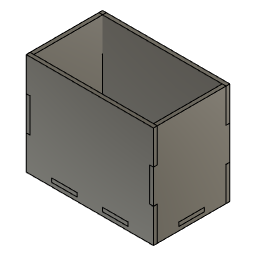
Parametric Box (Autodesk Fusion 360 design; units mm, degrees)
Autodesk Fusion 360 part; units mm, degrees
sketch "Sketch1" plane through (0, 0, 0) normal (0, 1, 0) x (1, 0, 0) in component "front"
  line L0 (0, 0) -> (100, 0)
  line L1 (100, 0) -> (100, -80)
  line L2 (100, -80) -> (0, -80)
  line L3 (0, -80) -> (0, 0)
  line L4 (3, 0) -> (3, -80) construction
  line L5 (0, -6) -> (100, -6) construction
  line L6 (100, -3) -> (0, -3) construction
  line L7 (50, -80) -> (50, 0) construction
  line L8 (20, -6) -> (40, -6)
  line L9 (40, -6) -> (40, -3)
  line L10 (40, -3) -> (20, -3)
  line L11 (20, -3) -> (20, -6)
  line L12 (60, -6) -> (80, -6)
  line L13 (80, -6) -> (80, -3)
  line L14 (80, -3) -> (60, -3)
  line L15 (60, -3) -> (60, -6)
  line L16 (0, -53.3333) -> (3, -53.3333)
  line L17 (3, -53.3333) -> (3, -26.6667)
  line L18 (3, -26.6667) -> (0, -26.6667)
  line L19 (0, -26.6667) -> (0, -53.3333)
  line L20 (100, -53.3333) -> (97, -53.3333)
  line L21 (100, -80) -> (100, 0)
  line L22 (97, -26.6667) -> (100, -26.6667)
  line L23 (97, 0) -> (97, -80) construction
  line L24 (100, -26.6667) -> (100, -53.3333)
  line L25 (97, -53.3333) -> (97, -26.6667)
  dimension "d10" = 100
  dimension "d11" = 80
  dimension "d12" = 3
  dimension "d13" = 3
  dimension "d14" = 3
  dimension "d17" = 20
  dimension "d18" = 20
  dimension "d19" = 20
  dimension "d20" = 20
  dimension "d21" = 26.6667
  dimension "d22" = 26.6667
  constraint horizontal L0
  constraint vertical L1
  constraint horizontal L2
  constraint vertical L3
  constraint coincident L0.start L3.end
  constraint coincident L0 L4.start
  constraint coincident L2 L4.end
  constraint perpendicular L2 L4
  constraint coincident L3 L5.start
  constraint coincident L1 L5.end
  constraint perpendicular L1 L5
  constraint coincident L1 L6.start
  constraint perpendicular L3 L6
  constraint coincident L3 L6.end
  constraint midpoint L2 L7.start
  constraint perpendicular L5 L7
  constraint horizontal L8
  constraint vertical L9
  constraint horizontal L10
  constraint vertical L11
  constraint coincident L6 L9.end
  constraint coincident L5 L8.start
  constraint horizontal L12
  constraint vertical L13
  constraint horizontal L14
  constraint vertical L15
  constraint coincident L6 L13.end
  constraint coincident L5 L12.start
  constraint horizontal L16
  constraint vertical L17
  constraint horizontal L18
  constraint vertical L19
  constraint coincident L4 L17.end
  constraint coincident L3 L16.start
  constraint symmetric L0.start L7 L0.end
  constraint symmetric L2.end L7 L1.end
  constraint symmetric L4.start L7 L23.start
  constraint symmetric L4.end L7 L23.end
  constraint symmetric L7 L16.start L20.start
  constraint symmetric L7 L16.end L20.end
  constraint symmetric L7 L17.end L22.start
  constraint symmetric L7 L18.end L22.end
  measures "d10" distance of L0.start L0.end
  measures "d11" distance of L0.start L2.end
  measures "d12" distance of L0 L6
  measures "d13" distance of L5 L6
  measures "d14" distance of L3 L4
  measures "d17" distance of L3 L8.start
  measures "d18" distance of L9.end L10.end
  measures "d19" distance of L9.end L14.end
  measures "d20" distance of L13.end L14.end
  measures "d21" distance of L2 L16
  measures "d22" distance of L16 L18
extrude "Extrude1" add sketch "Sketch1" along normal blind 3 contours L0 L1 L2 L3 L16 L17 L18 L20 L21 L22 L25 makes body 1 in component "front"
sketch "Sketch1 (2)" plane through (0, 0, 0) normal (1, 0, 0) x (0, 1, 0) in component "left"
sketch "Sketch2" plane through (0, 0, 0) normal (1, 0, 0) x (0, 1, 0) in component "left"
  line L0 (0, 0) -> (60, 0)
  line L1 (60, 0) -> (60, 80)
  line L2 (60, 80) -> (0, 80)
  line L3 (0, 80) -> (0, 0)
  line L4 (0, 80) -> (0, 53.3333)
  line L5 (0, 80) -> (3, 80)
  line L6 (0, 0) -> (3, 0)
  line L7 (0, 6) -> (60, 6) construction
  line L8 (0, 3) -> (60, 3) construction
  line L9 (40, 6) -> (20, 6)
  line L10 (20, 6) -> (20, 3)
  line L11 (20, 3) -> (40, 3)
  line L12 (40, 3) -> (40, 6)
  dimension "d25" = 60
  dimension "d26" = 20
  dimension "d27" = 20
  dimension "d28" = 3
  dimension "d29" = 3
  constraint horizontal L0
  constraint vertical L1
  constraint horizontal L2
  constraint vertical L3
  constraint collinear L3 L4
  constraint collinear L2 L5
  constraint collinear L0 L6
  constraint coincident L3 L7.start
  constraint coincident L1 L7.end
  constraint perpendicular L1 L7
  constraint coincident L3 L8.start
  constraint coincident L1 L8.end
  constraint perpendicular L1 L8
  constraint horizontal L9
  constraint vertical L10
  constraint horizontal L11
  constraint vertical L12
  constraint coincident L7 L9.start
  measures "d25" distance of L1 L3
  measures "d26" distance of L9.start L9.end
  measures "d27" distance of L1 L12
  measures "d28" distance of L7 L8
  measures "d29" distance of L0 L8
extrude "Extrude1'" add sketch "Sketch2" along normal blind 3 separate body makes body 2 in component "left"
combine "Combine1" operation cut target body 2 tool bodies 1 keep tools in component "left"
ref_plane "WorkPlane1" through (50, 1.5, 66.6667) normal (-1, 0, 0) x (0, 0, 1)
mirror "MirrorComponent1" about plane through (0, 0, 0) normal (0, 0, 1) of bodies 2 makes body 3 in component "left(Mirror)"
ref_plane "WorkPlane2" through (1.5, 30, 40) normal (0, 1, 0) x (0, 0, 1)
mirror "MirrorComponent2" about plane through (0, 0, 0) normal (0, 0, 1) of bodies 1 makes body 4 in component "front(Mirror)"
combine "Combine1'" operation cut target body 3 tool bodies 4 body 4 seen with x (-1, 0, 0) y (0, -1, 0) z (0, 0, 1) at (100, 60, 0) keep tools in component "left(Mirror)"
ref_plane "WorkPlane1" through (0, 0, 3) normal (0, 0, 1) x (1, 0, 0) in component "base"
sketch "Sketch1 (3)" plane through (0, 0, 3) normal (0, 0, 1) x (1, 0, 0) in component "base"
  line L0 (0, 60) -> (100, 60)
  line L1 (100, 60) -> (100, 0)
  line L2 (100, 0) -> (0, 0)
  line L3 (0, 0) -> (0, 60)
  constraint horizontal L0
  constraint vertical L1
  constraint horizontal L2
  constraint vertical L3
extrude "Extrude1''" add sketch "Sketch1 (3)" along normal blind 3 separate body makes body 5 in component "base"
combine "Combine1''" operation cut target body 5 tool bodies 2 4 3 1 body 4 seen with x (1, 0, 0) y (0, -1, 0) z (0, 0, -1) at (0, 60, 0) body 3 seen with x (-1, 0, 0) y (0, 1, 0) z (0, 0, -1) at (100, 0, 0) keep tools in component "base"
component "front" placed x (1, 0, 0) y (0, 1, 0) z (0, 0, 1) at (0, 0, 0)
component "left" placed x (1, 0, 0) y (0, 1, 0) z (0, 0, 1) at (0, 0, 0)
component "left(Mirror)" placed x (-1, 0, 0) y (0, 1, 0) z (0, 0, -1) at (100, 0, 0)
component "front(Mirror)" placed x (1, 0, 0) y (0, -1, 0) z (0, 0, -1) at (0, 60, 0)
component "base" placed x (1, 0, 0) y (0, 1, 0) z (0, 0, 1) at (0, 0, 0)
equation "length = 100 mm"
equation "width = 60 mm"
equation "height = 80 mm"
equation "thick = 3 mm"
equation "ntabs_L = 5"
equation "ntabs_W = 3"
equation "ntabs_H = 3"
equation "d10 = length"
equation "d11 = height"
equation "d12 = thick"
equation "d13 = thick"
equation "d14 = thick"
equation "d15 = length / ntabs_L"
equation "d16 = d15"
equation "d17 = d16"
equation "d18 = d17"
equation "d19 = d18"
equation "d21 = height / ntabs_H"
equation "d22 = d21"
equation "d23 = thick"
equation "d25 = width"
equation "d26 = width / ntabs_W"
equation "d27 = d26"
equation "d28 = thick"
equation "d29 = thick"
equation "d30 = thick"
equation "d32 = thick"
equation "d33 = thick"
